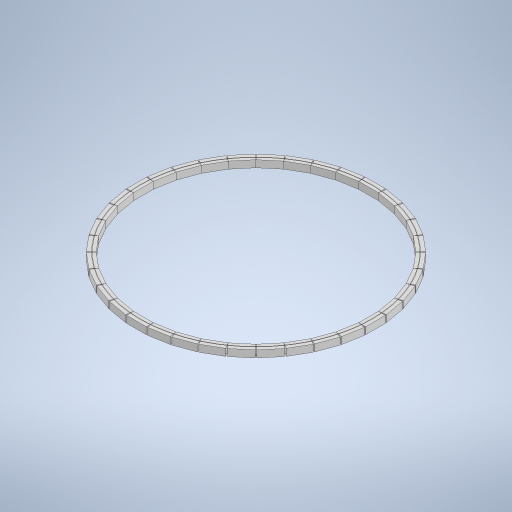
# Autodesk Inventor part: 柱-1 磚-2
Saved by Autodesk Inventor 2024 (Build 280153000, 153)
## iProperties
Created: 2024-05-18
Part Number: 柱-1 磚-2
Material: 一般
Document SubType Name: Modeling
Designer: User
Density: 1 g/cm^3
Appearance: 預設
Author: User
Autodesk Inventor part; units mm, degrees
ref_plane "YZ Plane" through (0, 0, 0) normal (1, 0, 0) x (0, 1, 0)
ref_plane "XZ Plane" through (0, 0, 0) normal (0, 1, 0) x (-1, 0, 0)
ref_plane "XY Plane" through (0, 0, 0) normal (0, 0, 1) x (1, 0, 0)
sketch "草圖1" plane through (0, 0, 0) normal (0, 1, 0) x (-1, 0, 0)
  circle A0 centre (0, 0) radius 25
  line L0 (24.25, 2.125) -> (25.75, 2.125)
  line L1 (25.75, 2.125) -> (25.75, -2.125)
  line L2 (25.75, -2.125) -> (24.25, -2.125)
  line L3 (24.25, -2.125) -> (24.25, 2.125)
  line L4 (24.25, 2.125) -> (25.75, -2.125) construction
  line L5 (25.75, 2.125) -> (24.25, -2.125) construction
  line L6 (24.9898, 6.5642) -> (25.7278, 2.3787)
  line L7 (23.5126, 6.3037) -> (24.9898, 6.5642)
  line L8 (24.2506, 2.1183) -> (23.5126, 6.3037)
  line L9 (25.7278, 2.3787) -> (24.2506, 2.1183)
  line L10 (23.4703, 10.8039) -> (24.9239, 6.8102)
  line L11 (22.0608, 10.2908) -> (23.4703, 10.8039)
  line L12 (23.5143, 6.2971) -> (22.0608, 10.2908)
  line L13 (24.9239, 6.8102) -> (23.5143, 6.2971)
  line L14 (21.2377, 14.7153) -> (23.3627, 11.0347)
  line L15 (19.9386, 13.9653) -> (21.2377, 14.7153)
  line L16 (22.0636, 10.2847) -> (19.9386, 13.9653)
  line L17 (23.3627, 11.0347) -> (22.0636, 10.2847)
  line L18 (18.3597, 18.1796) -> (21.0916, 14.9239)
  line L19 (17.2107, 17.2154) -> (18.3597, 18.1796)
  line L20 (19.9425, 13.9598) -> (17.2107, 17.2154)
  line L21 (21.0916, 14.9239) -> (19.9425, 13.9598)
  line L22 (14.9239, 21.0916) -> (18.1796, 18.3597)
  line L23 (13.9598, 19.9425) -> (14.9239, 21.0916)
  line L24 (17.2154, 17.2107) -> (13.9598, 19.9425)
  line L25 (18.1796, 18.3597) -> (17.2154, 17.2107)
  line L26 (11.0347, 23.3627) -> (14.7153, 21.2377)
  line L27 (10.2847, 22.0636) -> (11.0347, 23.3627)
  line L28 (13.9653, 19.9386) -> (10.2847, 22.0636)
  line L29 (14.7153, 21.2377) -> (13.9653, 19.9386)
  line L30 (6.8102, 24.9239) -> (10.8039, 23.4703)
  line L31 (6.2971, 23.5143) -> (6.8102, 24.9239)
  line L32 (10.2908, 22.0608) -> (6.2971, 23.5143)
  line L33 (10.8039, 23.4703) -> (10.2908, 22.0608)
  line L34 (2.3787, 25.7278) -> (6.5642, 24.9898)
  line L35 (2.1183, 24.2506) -> (2.3787, 25.7278)
  line L36 (6.3037, 23.5126) -> (2.1183, 24.2506)
  line L37 (6.5642, 24.9898) -> (6.3037, 23.5126)
  line L38 (-2.125, 25.75) -> (2.125, 25.75)
  line L39 (-2.125, 24.25) -> (-2.125, 25.75)
  line L40 (2.125, 24.25) -> (-2.125, 24.25)
  line L41 (2.125, 25.75) -> (2.125, 24.25)
  line L42 (-6.5642, 24.9898) -> (-2.3787, 25.7278)
  line L43 (-6.3037, 23.5126) -> (-6.5642, 24.9898)
  line L44 (-2.1183, 24.2506) -> (-6.3037, 23.5126)
  line L45 (-2.3787, 25.7278) -> (-2.1183, 24.2506)
  line L46 (-10.8039, 23.4703) -> (-6.8102, 24.9239)
  line L47 (-10.2908, 22.0608) -> (-10.8039, 23.4703)
  line L48 (-6.2971, 23.5143) -> (-10.2908, 22.0608)
  line L49 (-6.8102, 24.9239) -> (-6.2971, 23.5143)
  line L50 (-14.7153, 21.2377) -> (-11.0347, 23.3627)
  line L51 (-13.9653, 19.9386) -> (-14.7153, 21.2377)
  line L52 (-10.2847, 22.0636) -> (-13.9653, 19.9386)
  line L53 (-11.0347, 23.3627) -> (-10.2847, 22.0636)
  line L54 (-18.1796, 18.3597) -> (-14.9239, 21.0916)
  line L55 (-17.2154, 17.2107) -> (-18.1796, 18.3597)
  line L56 (-13.9598, 19.9425) -> (-17.2154, 17.2107)
  line L57 (-14.9239, 21.0916) -> (-13.9598, 19.9425)
  line L58 (-21.0916, 14.9239) -> (-18.3597, 18.1796)
  line L59 (-19.9425, 13.9598) -> (-21.0916, 14.9239)
  line L60 (-17.2107, 17.2154) -> (-19.9425, 13.9598)
  line L61 (-18.3597, 18.1796) -> (-17.2107, 17.2154)
  line L62 (-23.3627, 11.0347) -> (-21.2377, 14.7153)
  line L63 (-22.0636, 10.2847) -> (-23.3627, 11.0347)
  line L64 (-19.9386, 13.9653) -> (-22.0636, 10.2847)
  line L65 (-21.2377, 14.7153) -> (-19.9386, 13.9653)
  line L66 (-24.9239, 6.8102) -> (-23.4703, 10.8039)
  line L67 (-23.5143, 6.2971) -> (-24.9239, 6.8102)
  line L68 (-22.0608, 10.2908) -> (-23.5143, 6.2971)
  line L69 (-23.4703, 10.8039) -> (-22.0608, 10.2908)
  line L70 (-25.7278, 2.3787) -> (-24.9898, 6.5642)
  line L71 (-24.2506, 2.1183) -> (-25.7278, 2.3787)
  line L72 (-23.5126, 6.3037) -> (-24.2506, 2.1183)
  line L73 (-24.9898, 6.5642) -> (-23.5126, 6.3037)
  line L74 (-25.75, -2.125) -> (-25.75, 2.125)
  line L75 (-24.25, -2.125) -> (-25.75, -2.125)
  line L76 (-24.25, 2.125) -> (-24.25, -2.125)
  line L77 (-25.75, 2.125) -> (-24.25, 2.125)
  line L78 (-24.9898, -6.5642) -> (-25.7278, -2.3787)
  line L79 (-23.5126, -6.3037) -> (-24.9898, -6.5642)
  line L80 (-24.2506, -2.1183) -> (-23.5126, -6.3037)
  line L81 (-25.7278, -2.3787) -> (-24.2506, -2.1183)
  line L82 (-23.4703, -10.8039) -> (-24.9239, -6.8102)
  line L83 (-22.0608, -10.2908) -> (-23.4703, -10.8039)
  line L84 (-23.5143, -6.2971) -> (-22.0608, -10.2908)
  line L85 (-24.9239, -6.8102) -> (-23.5143, -6.2971)
  line L86 (-21.2377, -14.7153) -> (-23.3627, -11.0347)
  line L87 (-19.9386, -13.9653) -> (-21.2377, -14.7153)
  line L88 (-22.0636, -10.2847) -> (-19.9386, -13.9653)
  line L89 (-23.3627, -11.0347) -> (-22.0636, -10.2847)
  line L90 (-18.3597, -18.1796) -> (-21.0916, -14.9239)
  line L91 (-17.2107, -17.2154) -> (-18.3597, -18.1796)
  line L92 (-19.9425, -13.9598) -> (-17.2107, -17.2154)
  line L93 (-21.0916, -14.9239) -> (-19.9425, -13.9598)
  line L94 (-14.9239, -21.0916) -> (-18.1796, -18.3597)
  line L95 (-13.9598, -19.9425) -> (-14.9239, -21.0916)
  line L96 (-17.2154, -17.2107) -> (-13.9598, -19.9425)
  line L97 (-18.1796, -18.3597) -> (-17.2154, -17.2107)
  line L98 (-11.0347, -23.3627) -> (-14.7153, -21.2377)
  line L99 (-10.2847, -22.0636) -> (-11.0347, -23.3627)
  line L100 (-13.9653, -19.9386) -> (-10.2847, -22.0636)
  line L101 (-14.7153, -21.2377) -> (-13.9653, -19.9386)
  line L102 (-6.8102, -24.9239) -> (-10.8039, -23.4703)
  line L103 (-6.2971, -23.5143) -> (-6.8102, -24.9239)
  line L104 (-10.2908, -22.0608) -> (-6.2971, -23.5143)
  line L105 (-10.8039, -23.4703) -> (-10.2908, -22.0608)
  line L106 (-2.3787, -25.7278) -> (-6.5642, -24.9898)
  line L107 (-2.1183, -24.2506) -> (-2.3787, -25.7278)
  line L108 (-6.3037, -23.5126) -> (-2.1183, -24.2506)
  line L109 (-6.5642, -24.9898) -> (-6.3037, -23.5126)
  line L110 (2.125, -25.75) -> (-2.125, -25.75)
  line L111 (2.125, -24.25) -> (2.125, -25.75)
  line L112 (-2.125, -24.25) -> (2.125, -24.25)
  line L113 (-2.125, -25.75) -> (-2.125, -24.25)
  line L114 (6.5642, -24.9898) -> (2.3787, -25.7278)
  line L115 (6.3037, -23.5126) -> (6.5642, -24.9898)
  line L116 (2.1183, -24.2506) -> (6.3037, -23.5126)
  line L117 (2.3787, -25.7278) -> (2.1183, -24.2506)
  line L118 (10.8039, -23.4703) -> (6.8102, -24.9239)
  line L119 (10.2908, -22.0608) -> (10.8039, -23.4703)
  line L120 (6.2971, -23.5143) -> (10.2908, -22.0608)
  line L121 (6.8102, -24.9239) -> (6.2971, -23.5143)
  line L122 (14.7153, -21.2377) -> (11.0347, -23.3627)
  line L123 (13.9653, -19.9386) -> (14.7153, -21.2377)
  line L124 (10.2847, -22.0636) -> (13.9653, -19.9386)
  line L125 (11.0347, -23.3627) -> (10.2847, -22.0636)
  line L126 (18.1796, -18.3597) -> (14.9239, -21.0916)
  line L127 (17.2154, -17.2107) -> (18.1796, -18.3597)
  line L128 (13.9598, -19.9425) -> (17.2154, -17.2107)
  line L129 (14.9239, -21.0916) -> (13.9598, -19.9425)
  line L130 (21.0916, -14.9239) -> (18.3597, -18.1796)
  line L131 (19.9425, -13.9598) -> (21.0916, -14.9239)
  line L132 (17.2107, -17.2154) -> (19.9425, -13.9598)
  line L133 (18.3597, -18.1796) -> (17.2107, -17.2154)
  line L134 (23.3627, -11.0347) -> (21.2377, -14.7153)
  line L135 (22.0636, -10.2847) -> (23.3627, -11.0347)
  line L136 (19.9386, -13.9653) -> (22.0636, -10.2847)
  line L137 (21.2377, -14.7153) -> (19.9386, -13.9653)
  line L138 (24.9239, -6.8102) -> (23.4703, -10.8039)
  line L139 (23.5143, -6.2971) -> (24.9239, -6.8102)
  line L140 (22.0608, -10.2908) -> (23.5143, -6.2971)
  line L141 (23.4703, -10.8039) -> (22.0608, -10.2908)
  line L142 (25.7278, -2.3787) -> (24.9898, -6.5642)
  line L143 (24.2506, -2.1183) -> (25.7278, -2.3787)
  line L144 (23.5126, -6.3037) -> (24.2506, -2.1183)
  line L145 (24.9898, -6.5642) -> (23.5126, -6.3037)
  point P0 (25, 0)
  point P1 (24.2889, 2.125)
  point P2 (23.5509, 6.3104)
  point P3 (22.0973, 10.3041)
  point P4 (19.9723, 13.9847)
  point P5 (17.2404, 17.2404)
  point P6 (13.9847, 19.9723)
  point P7 (10.3041, 22.0973)
  point P8 (6.3104, 23.5509)
  point P9 (2.125, 24.2889)
  point P10 (-2.125, 24.2889)
  point P11 (-6.3104, 23.5509)
  point P12 (-10.3041, 22.0973)
  point P13 (-13.9847, 19.9723)
  point P14 (-17.2404, 17.2404)
  point P15 (-19.9723, 13.9847)
  point P16 (-22.0973, 10.3041)
  point P17 (-23.5509, 6.3104)
  point P18 (-24.2889, 2.125)
  point P19 (-24.2889, -2.125)
  point P20 (-23.5509, -6.3104)
  point P21 (-22.0973, -10.3041)
  point P22 (-19.9723, -13.9847)
  point P23 (-17.2404, -17.2404)
  point P24 (-13.9847, -19.9723)
  point P25 (-10.3041, -22.0973)
  point P26 (-6.3104, -23.5509)
  point P27 (-2.125, -24.2889)
  point P28 (2.125, -24.2889)
  point P29 (6.3104, -23.5509)
  point P30 (10.3041, -22.0973)
  point P31 (13.9847, -19.9723)
  point P32 (17.2404, -17.2404)
  point P33 (19.9723, -13.9847)
  point P34 (22.0973, -10.3041)
  point P35 (23.5509, -6.3104)
  point P36 (24.2889, -2.125)
  point P37 (24.25, 2.1216)
  point P38 (24.25, -2.1216)
  point P39 (23.5132, -6.3003)
  point P40 (22.0619, -10.2876)
  point P41 (19.9403, -13.9624)
  point P42 (17.2128, -17.2128)
  point P43 (13.9624, -19.9403)
  point P44 (10.2876, -22.0619)
  point P45 (6.3003, -23.5132)
  point P46 (2.1216, -24.25)
  point P47 (-2.1216, -24.25)
  point P48 (-6.3003, -23.5132)
  point P49 (-10.2876, -22.0619)
  point P50 (-13.9624, -19.9403)
  point P51 (-17.2128, -17.2128)
  point P52 (-19.9403, -13.9624)
  point P53 (-22.0619, -10.2876)
  point P54 (-23.5132, -6.3003)
  point P55 (-24.25, -2.1216)
  point P56 (-24.25, 2.1216)
  point P57 (-23.5132, 6.3003)
  point P58 (-22.0619, 10.2876)
  point P59 (-19.9403, 13.9624)
  point P60 (-17.2128, 17.2128)
  point P61 (-13.9624, 19.9403)
  point P62 (-10.2876, 22.0619)
  point P63 (-6.3003, 23.5132)
  point P64 (-2.1216, 24.25)
  point P65 (2.1216, 24.25)
  point P66 (6.3003, 23.5132)
  point P67 (10.2876, 22.0619)
  point P68 (13.9624, 19.9403)
  point P69 (17.2128, 17.2128)
  point P70 (19.9403, 13.9624)
  point P71 (22.0619, 10.2876)
  point P72 (23.5132, 6.3003)
  dimension "d0" = 50
  dimension "d1" = 1.5
  dimension "d2" = 4.25
  dimension "d5" = 360
  constraints: 292 end point, 2 midpoint, 2 parallel, 1 coincident, 1 horizontal, 1 horizontal alignment, 1 perpendicular, 291 other
  measures "d1" distance of L1.end L2.end
  measures "d2" distance of L0.end L1.end
extrude "擠出1" add sketch "草圖1" along normal blind 1.5 contours A0 L2 L143 L3 L9 L0 | A0 L0 L1 L2 | L9 L0 L8 L13 L7 A0 | A0 L7 L6 L9 | L9 L3 L0 | L143 L142 L145 A0 | A0 L145 L139 L144 L2 L143 | L2 L3 L143 | L13 L7 L12 L17 L11 A0 | A0 L11 L10 L13 | L13 L8 L7 | L139 L138 L141 A0 | A0 L141 L135 L140 L145 L139 | L145 L140 L139 | L17 L11 L16 L21 L15 A0 | A0 L15 L14 L17 | L17 L12 L11 | L135 L134 L137 A0 | A0 L137 L131 L136 L141 L135 | L141 L136 L135 | L21 L15 L20 L25 L19 A0 | A0 L19 L18 L21 | L21 L16 L15 | L131 L130 L133 A0 | A0 L133 L127 L132 L137 L131 | L137 L132 L131 | L25 L19 L24 L29 L23 A0 | A0 L23 L22 L25 | L25 L20 L19 | L127 L126 L129 A0 | A0 L129 L123 L128 L133 L127 | L133 L128 L127 | L29 L23 L28 L33 L27 A0 | A0 L27 L26 L29 | L29 L24 L23 | L123 L122 L125 A0 | A0 L125 L119 L124 L129 L123 | L129 L124 L123 | L33 L27 L32 L37 L31 A0 | A0 L31 L30 L33 | L33 L28 L27 | L119 L118 L121 A0 | A0 L121 L115 L120 L125 L119 | L125 L120 L119 | L37 L31 L36 L41 L35 A0 | A0 L35 L34 L37 | L37 L32 L31 | L115 L114 L117 A0 | A0 L117 L111 L116 L121 L115 | L121 L116 L115 | L41 L35 L40 L45 L39 A0 | A0 L39 L38 L41 | L41 L36 L35 | L111 L110 L113 A0 | A0 L113 L107 L112 L117 L111 | L117 L112 L111 | L45 L39 L44 L49 L43 A0 | A0 L43 L42 L45 | L45 L40 L39 | L107 L106 L109 A0 | A0 L109 L103 L108 L113 L107 | L113 L108 L107 | L49 L43 L48 L53 L47 A0 | A0 L47 L46 L49 | L49 L44 L43 | L103 L102 L105 A0 | A0 L105 L99 L104 L109 L103 | L109 L104 L103 | L53 L47 L52 L57 L51 A0 | A0 L51 L50 L53 | L53 L48 L47 | L99 L98 L101 A0 | A0 L101 L95 L100 L105 L99 | L105 L100 L99 | L57 L51 L56 L61 L55 A0 | A0 L55 L54 L57 | L57 L52 L51 | L95 L94 L97 A0 | A0 L97 L91 L96 L101 L95 | L101 L96 L95 | L61 L55 L60 L65 L59 A0 | A0 L59 L58 L61 | L61 L56 L55 | L91 L90 L93 A0 | A0 L93 L87 L92 L97 L91 | L97 L92 L91 | L65 L59 L64 L69 L63 A0 | A0 L63 L62 L65 | L65 L60 L59 | L87 L86 L89 A0 | A0 L89 L83 L88 L93 L87 | L93 L88 L87 | L69 L63 L68 L73 L67 A0 | A0 L67 L66 L69 | L69 L64 L63 | L83 L82 L85 A0 | A0 L85 L79 L84 L89 L83 | L89 L84 L83 | L73 L67 L72 L77 L71 A0 | A0 L71 L70 L73 | L73 L68 L67 | L79 L78 L81 A0 | A0 L81 L75 L80 L85 L79 | L85 L80 L79 | L77 L71 L76 L81 L75 A0 | A0 L75 L74 L77 | L77 L72 L71 | L81 L76 L75
sketch "草圖2" plane through (0, 0, 0) normal (0, 1, 0) x (-1, 0, 0)
  circle A0 centre (0, 0) radius 24.95
  circle A1 centre (0, 0) radius 25.05
  dimension "d9" = 49.9
  dimension "d10" = 50.1
  constraints: 2 centre point, 2 coincident
  measures "d9" diameter of A0
  measures "d10" diameter of A1
extrude "擠出2" add sketch "草圖2" along normal blind 1.5 separate body
